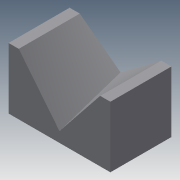
# Autodesk Inventor part: LoftCut
Saved by Autodesk Inventor 2015 (Build 190159000, 159)
## iProperties
Created: 2016-11-12
Part Number: LoftCut
Material: Generic
Document SubType Name: Modeling
Designer: Aniket Pant
Density: 1 g/cm^3
Appearance: Default
Author: Aniket Pant
Autodesk Inventor part; units mm, degrees
ref_plane "YZ Plane" through (0, 0, 0) normal (1, 0, 0) x (0, 1, 0)
ref_plane "XZ Plane" through (0, 0, 0) normal (0, 1, 0) x (-1, 0, 0)
ref_plane "XY Plane" through (0, 0, 0) normal (0, 0, 1) x (1, 0, 0)
sketch "Sketch1" plane through (0, 0, 0) normal (0, 0, 1) x (1, 0, 0)
  line L0 (10.2557, 10.2212) -> (73.7557, 10.2212)
  line L1 (73.7557, 10.2212) -> (73.7557, 48.3212)
  line L2 (73.7557, 48.3212) -> (10.2557, 48.3212)
  line L3 (10.2557, 48.3212) -> (10.2557, 10.2212)
  point P0 (0, 0)
  dimension "d0" = 63.5
  dimension "d1" = 38.1
  constraints: 8 end point, 2 parallel, 1 horizontal, 1 perpendicular
  measures "d0" distance of L2.end L1.end
  measures "d1" distance of L1.end L0.end
extrude "Extrusion1" add sketch "Sketch1" against normal blind 38.1
sketch "Sketch2" plane through (0, 0, 0) normal (0, 0, 1) x (1, 0, 0)
  line L0 (10.2557, 10.2212) -> (73.7557, 10.2212) projected
  line L1 (73.7557, 10.2212) -> (73.7557, 48.3212) projected
  line L2 (73.7557, 48.3212) -> (10.2557, 48.3212) projected
  line L3 (10.2557, 48.3212) -> (10.2557, 10.2212) projected
  line L4 (10.2557, 48.3212) -> (73.7557, 48.3212)
  line L5 (73.7557, 48.3212) -> (73.7557, 10.2212)
  line L6 (73.7557, 10.2212) -> (10.2557, 10.2212)
  line L7 (10.2557, 10.2212) -> (10.2557, 48.3212)
  line L8 (10.2557, 48.3212) -> (73.7557, 48.3212) projected
  line L9 (16.6057, 48.3212) -> (42.0057, 16.5712)
  line L10 (42.0057, 16.5712) -> (67.4057, 48.3212)
  point P0 (0, 0)
  dimension "d4" = 6.35
  dimension "d5" = 6.35
  dimension "d6" = 6.35
  constraints: 12 end point, 2 parallel, 2 point on line, 1 equal length, 1 horizontal, 1 perpendicular
  measures "d4" distance from line of L0 L9.end
  measures "d5" distance of L2.end L9.start
  measures "d6" distance of L1.end L10.end
sketch "Sketch3" plane through (0, 0, -38.1) normal (0, 0, -1) x (-1, 0, 0)
  line L0 (-73.7557, 10.2212) -> (-10.2557, 10.2212) projected
  line L1 (-10.2557, 10.2212) -> (-10.2557, 48.3212) projected
  line L2 (-10.2557, 48.3212) -> (-73.7557, 48.3212) projected
  line L3 (-73.7557, 48.3212) -> (-73.7557, 10.2212) projected
  line L4 (-73.7557, 48.3212) -> (-10.2557, 48.3212)
  line L5 (-10.2557, 48.3212) -> (-10.2557, 10.2212)
  line L6 (-10.2557, 10.2212) -> (-73.7557, 10.2212)
  line L7 (-73.7557, 10.2212) -> (-73.7557, 48.3212)
  line L8 (-10.2557, 48.3212) -> (-73.7557, 48.3212) projected
  line L9 (-67.4057, 48.3212) -> (-42.0057, 29.2712)
  line L10 (-42.0057, 29.2712) -> (-16.6057, 48.3212)
  point P0 (0, 0)
  dimension "d7" = 19.05
  dimension "d8" = 6.35
  dimension "d9" = 6.35
  constraints: 12 end point, 2 parallel, 2 point on line, 1 equal length, 1 horizontal, 1 perpendicular
  measures "d7" distance from line of L0 L9.end
  measures "d8" distance of L2.end L9.start
  measures "d9" distance of L1.end L10.end
loft "Loft1" cut profiles "Sketch2", "Sketch3" keep common part contours L3 L2 L9 L10 L1 L0 / L3 L2 L9 L10 L1 L0
equation "\"d6\" = d5"
body "Solid1"
